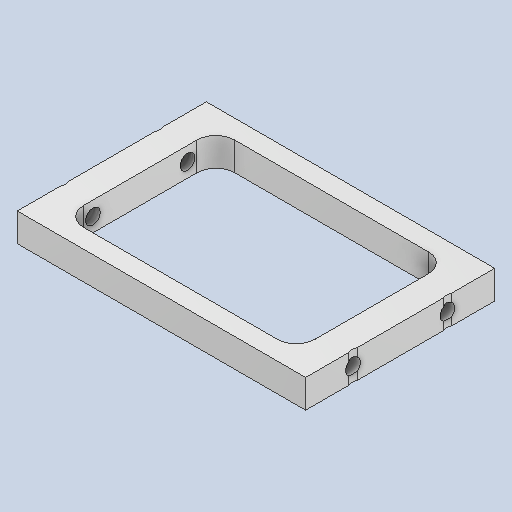
# Autodesk Inventor part: free_suzikai
Saved by Autodesk Inventor 2025.1 (Build 291241000, 241)
## iProperties
Created: 2024-09-02
Part Number: free_suzikai
Material: アルミニウム 2014-T4
Document SubType Name: Modeling
Designer: right
Density: 2.8 g/cm^3
Appearance: サテン
Mass: 1.79423 g
Surface Area: 10.2139 cm^2
Volume: 0.640795 cm^3
Author: right
Autodesk Inventor part; units mm, degrees
ref_plane "YZ Plane" through (0, 0, 0) normal (1, 0, 0) x (0, 1, 0)
ref_plane "XZ Plane" through (0, 0, 0) normal (0, 1, 0) x (-1, 0, 0)
ref_plane "XY Plane" through (0, 0, 0) normal (0, 0, 1) x (1, 0, 0)
sketch "スケッチ1" plane through (0, 0, 0) normal (0, 1, 0) x (-1, 0, 0)
  line L0 (15.25, 10) -> (-15.25, 10)
  line L1 (-15.25, 10) -> (-15.25, -10)
  line L2 (-15.25, -10) -> (15.25, -10)
  line L3 (15.25, -10) -> (15.25, 10)
  line L4 (15.25, 10) -> (-15.25, -10) construction
  line L5 (-15.25, 10) -> (15.25, -10) construction
  line L6 (12.25, -8) -> (-12.25, -8)
  line L7 (-12.25, -8) -> (-12.25, 8)
  line L8 (-12.25, 8) -> (12.25, 8)
  line L9 (12.25, 8) -> (12.25, -8)
  circle A0 centre (-16.25, -5) radius 1.1
  line L10 (-15.25, 0) -> (15.25, 0) construction
  line L11 (0, 0) -> (0, -10) construction
  circle A1 centre (-16.25, 5) radius 1.1
  circle A2 centre (16.25, -5) radius 1.1
  circle A3 centre (16.25, 5) radius 1.1
  point P0 (0, 0)
  point P1 (-15.25, 5.4583)
  point P2 (-15.25, 4.5417)
  point P3 (-15.25, -4.5417)
  point P4 (-15.25, -5.4583)
  point P5 (15.25, -5.4583)
  point P6 (15.25, -4.5417)
  point P7 (15.25, 4.5417)
  point P8 (15.25, 5.4583)
  dimension "d0" = 30.5
  dimension "d1" = 20
  dimension "d3" = 2.2
  dimension "d4" = 1
  dimension "d5" = 10
  dimension "d16" = 2
  dimension "d17" = 2
  dimension "d18" = 3
  dimension "d19" = 3
  constraints: 24 end point, 7 midpoint, 4 centre point, 4 parallel, 3 symmetric about line, 2 perpendicular, 1 horizontal, 3 other
  measures "d0" distance of L1.end L2.end
  measures "d1" distance of L0.end L1.end
  measures "d3" diameter of A0
  measures "d4" distance from line of L1 A0.centre
  measures "d5" distance of A1.centre A0.centre
  measures "d16" distance between parallel lines of L2 L6
  measures "d17" distance between parallel lines of L0 L8
  measures "d18" distance between parallel lines of L3 L9
  measures "d19" distance between parallel lines of L1 L7
extrude "押し出し1" add sketch "スケッチ1" along normal blind 3 contours L3 A3 A2 L2 L1 A0 A1 L0
fillet "フィレット1" radius 2 4 edges at (12.25, 1.5, -8) (12.25, 1.5, 8) (-12.25, 1.5, 8) (-12.25, 1.5, -8)
sketch "スケッチ2" plane through (-15.25, 0, -4.5417) normal (-1, 0, 0) x (0, 0, 1)
  line L0 (10.5417, 3) -> (10.5417, 0)
  line L1 (-1.4583, 0) -> (-1.4583, 3)
  line L2 (-1.4583, 3) -> (-1.4583, 0)
  line L3 (-0.9165, 0) -> (0, 0)
  line L4 (-1.4583, 3) -> (-1.4583, 0) projected
  line L5 (-0.9165, 0) -> (0, 0) projected
  line L6 (9.0835, 0) -> (10, 0) projected
  line L7 (10.5417, 0) -> (10.5417, 3) projected
  point P0 (4.5417, 0)
  point P1 (9.5417, 1.5)
  point P2 (-0.4583, 1.5)
  point P3 (-1.4583, 1.5)
  point P4 (-0.4583, 0)
  point P5 (9.5417, 0)
  point P6 (10.5417, 1.5)
  constraints: 6 end point, 4 midpoint, 2 horizontal alignment, 2 vertical alignment, 3 other
hole "穴1" at (-15.25, 1.5, 5) at (-15.25, 1.5, -5) direction (1, 0, 0) diameter 1.567 end through all thread size "M2x0.4" class "6H" standard "ISO Metric profile"
equation "\"d17\" = d16"
equation "\"d19\" = d18"
